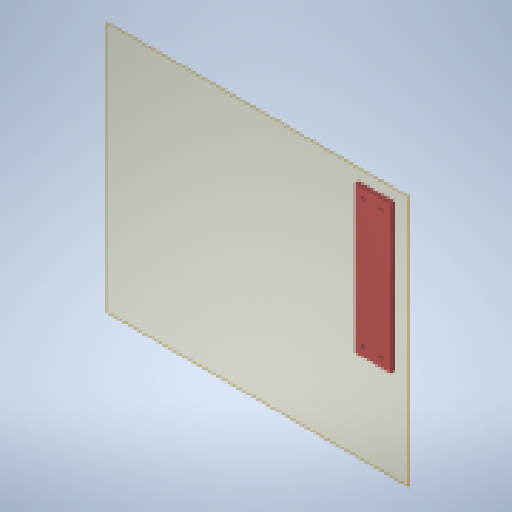
# Autodesk Inventor part: ReposadorPinzas
Saved by Autodesk Inventor 2023.1 (Build 271208000, 208)
## iProperties
Created: 2022-11-01
Part Number: ReposadorPinzas
Material: MDF Medium Density Fiberboard
Document SubType Name: Modeling
Designer: Daniel Peña
Density: 0.8 g/cm^3
Appearance: Chestnut
Author: Daniel Peña
Autodesk Inventor part; units mm, degrees
ref_plane "YZ Plane" through (0, 0, 0) normal (1, 0, 0) x (0, 1, 0)
ref_plane "XZ Plane" through (0, 0, 0) normal (0, 1, 0) x (-1, 0, 0)
ref_plane "XY Plane" through (0, 0, 0) normal (0, 0, 1) x (1, 0, 0)
sketch "Sketch1" plane through (0, 0, 0) normal (0, 0, 1) x (1, 0, 0)
  line L0 (150, 125) -> (110, 125)
  line L1 (110, 125) -> (110, -35)
  line L2 (110, -35) -> (150, -35)
  line L3 (150, -35) -> (150, 125)
  point P0 (0, 0)
  dimension "d0" = 40
  dimension "d3" = 160
  constraints: 8 end point, 2 parallel, 1 horizontal, 1 perpendicular
  measures "d0" distance of L2.end L1.end
  measures "d3" distance of L2.end L0.start
extrude "Extrusion1" add sketch "Sketch1" along normal blind 5
ref_plane "Work Plane1" through (0, 0, 0) normal (0, 0, 1) x (1, 0, 0)
sketch "Sketch3" plane through (0, 0, 5) normal (0, 0, 1) x (1, 0, 0)
  line L0 (150, 125) -> (110, 125) construction
  line L1 (130, 125) -> (130, -35) construction
  line L2 (110, -35) -> (150, -35) construction
  line L3 (110, 125) -> (110, -35) construction
  line L4 (110, 45) -> (150, 45) construction
  line L5 (150, -35) -> (150, 125) construction
  point P0 (0, 0)
  point P1 (120, 115)
  point P2 (140, 115)
  point P3 (120, -25)
  point P4 (140, -25)
  dimension "d4" = 20
  dimension "d5" = 10
  constraints: 4 end point, 4 midpoint, 3 symmetric about line
  measures "d4" distance of point (140, 115) point (120, 115)
  measures "d5" distance from line of L0 point (120, 115)
hole "Hole1" at (120, 115, 5) at (140, 115, 5) at (120, -25, 5) at (140, -25, 5) direction (0, 0, -1) diameter 5 end through all
body "Solid1"
